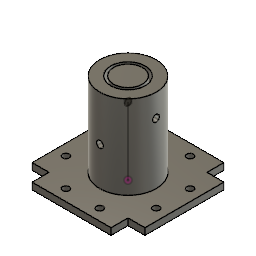
_pend_connector.6113d6a6-ff1e-4e22-9ab8-4d74f2541897 (Autodesk Fusion 360 design; units mm, degrees)
Autodesk Fusion 360 part; units mm, degrees
sketch "Sketch1" plane through (0, 0, 0) normal (0, 1, 0) x (1, 0, 0)
  line L0 (17.5, 25) -> (-17.5, 25)
  line L1 (-17.5, 25) -> (-17.5, -25)
  line L2 (-17.5, -25) -> (17.5, -25)
  line L3 (17.5, -25) -> (17.5, 25)
  line L4 (17.5, 25) -> (-17.5, -25) construction
  line L5 (-17.5, 25) -> (17.5, -25) construction
  line L6 (25, 17.5) -> (-25, 17.5)
  line L7 (-25, 17.5) -> (-25, -17.5)
  line L8 (-25, -17.5) -> (25, -17.5)
  line L9 (25, -17.5) -> (25, 17.5)
  line L10 (25, 17.5) -> (-25, -17.5) construction
  line L11 (-25, 17.5) -> (25, -17.5) construction
  circle A0 centre (0, 0) radius 7.6
  circle A1 centre (0, 0) radius 6.4
  circle A2 centre (0, 0) radius 12.5
  circle A3 centre (-20, 7.5) radius 1.5
  circle A4 centre (-20, -7.5) radius 1.5
  circle A5 centre (-7.5, -20) radius 1.5
  circle A6 centre (7.5, -20) radius 1.5
  circle A7 centre (20, -7.5) radius 1.5
  circle A8 centre (20, 7.5) radius 1.5
  circle A9 centre (7.5, 20) radius 1.5
  circle A10 centre (-7.5, 20) radius 1.5
  dimension "d1" = 50
  dimension "d2" = 35
  dimension "d3" = 50
  dimension "d4" = 35
  dimension "d5" = 15.2
  dimension "d6" = 12.8
  dimension "d7" = 25
  dimension "d8" = 3
  dimension "d9" = 3
  dimension "d10" = 10
  dimension "d11" = 10
  dimension "d12" = 5
  dimension "d13" = 5
  dimension "d15" = 360
  measures "d1" distance of L0.end L1.end
  measures "d2" distance of L1.end L2.end
  measures "d3" distance of L7.end L8.end
  measures "d4" distance of L6.end L7.end
  measures "d5" diameter of A0
  measures "d6" diameter of A1
  measures "d7" diameter of A2
  measures "d8" diameter of A3
  measures "d9" diameter of A4
  measures "d10" distance of L8 A4.centre
  measures "d11" distance of L6 A3.centre
  measures "d12" distance of L7 A3.centre
  measures "d13" distance of L7 A4.centre
extrude "Extrude1" add sketch "Sketch1" along normal blind 3 contours L0 L1 L3 L6 | L3 L6 L8 L9 | L1 L3 L6 L8 | L1 L6 L7 L8 | L1 L2 L3 L8 makes body 1
extrude "Extrude2" add sketch "Sketch1" along normal blind 10 separate body contours A0 makes body 2
extrude "Extrude3" add sketch "Sketch1" along normal blind 40 contours A1 | A2 bodies 1 2
sketch "Sketch2" plane through (0, 10, 0) normal (0, 1, 0) x (-1, 0, 0)
  circle A0 centre (0, 0) radius 6.4
  circle A1 centre (0, 0) radius 7.6
sketch "Sketch4" plane through (0, 0, 0) normal (0, 0, 1) x (1, 0, 0)
  circle A0 centre (0, 20) radius 1.5
  line L0 (0, 20) -> (0, 0)
  dimension "d22" = 3
  dimension "d23" = 20
  measures "d22" diameter of A0
  measures "d23" distance of A0.centre L0.end
extrude "Extrude4" cut sketch "Sketch4" against normal blind 30 bodies 1
extrude "Extrude5" cut sketch "Sketch4" along normal blind 30 bodies 1
sketch "Sketch6" plane through (0, 0, 0) normal (1, 0, 0) x (0, 0, -1)
  circle A0 centre (0, 30) radius 1.5
  line L0 (0, 30) -> (0, 0)
  dimension "d28" = 3
  dimension "d29" = 30
  measures "d28" diameter of A0
  measures "d29" distance of A0.centre L0.end
extrude "Extrude6" cut sketch "Sketch6" against normal blind 30 bodies 1
extrude "Extrude7" cut sketch "Sketch6" along normal blind 30 bodies 1
sketch "Sketch7" plane through (0, 0, 0) normal (0, 1, 0) x (1, 0, 0)
  circle A0 centre (0, 0) radius 1
  dimension "d34" = 2
  measures "d34" diameter of A0
extrude "Extrude8" cut sketch "Sketch7" along normal blind 10 bodies 1
